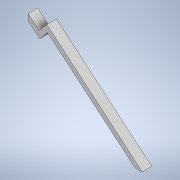
# Autodesk Inventor part: newFrame1x2piecsV03
Saved by Autodesk Inventor 2020.2 (Build 242310000, 310)
## iProperties
Created: 2020-02-22
Part Number: newFrame1x2piecsV03
Material: Generic
Document SubType Name: Modeling
Designer: robst
Density: 1 g/cm^3
Appearance: Default
Author: robst
Autodesk Inventor part; units mm, degrees
ref_plane "YZ Plane" through (0, 0, 0) normal (1, 0, 0) x (0, 1, 0)
ref_plane "XZ Plane" through (0, 0, 0) normal (0, 1, 0) x (-1, 0, 0)
ref_plane "XY Plane" through (0, 0, 0) normal (0, 0, 1) x (1, 0, 0)
sketch "Sketch1" plane through (0, 0, 0) normal (0, 0, 1) x (1, 0, 0)
  line L0 (0, 0) -> (-505.8958, 424.4969)
  line L1 (0, 0) -> (-228.6, 0) construction
  line L2 (0, 0) -> (-39.5154, 0)
  line L3 (-39.5154, 0) -> (-502.765, 388.7126)
  line L4 (-505.8958, 424.4969) -> (-522.2226, 405.0394)
  line L5 (-522.2226, 405.0394) -> (-546.7128, 375.8531)
  line L6 (-527.2552, 359.5263) -> (-502.765, 388.7126)
  line L7 (-546.7128, 375.8531) -> (-605.0854, 424.8335)
  line L8 (-605.0854, 391.6762) -> (-563.0396, 356.3956)
  line L9 (-543.582, 340.0688) -> (-527.2552, 359.5263)
  line L10 (-563.0396, 356.3956) -> (-543.582, 340.0688)
  line L11 (-228.6, 0) -> (-203.2, 0)
  line L12 (-605.0854, 424.8335) -> (-605.0854, 391.6762)
  line L13 (0, 0) -> (0, 391.6762) construction
  dimension "d2" = 660.4
  dimension "d3" = 25.4
  dimension "d4" = 40
  dimension "d25" = 50
  dimension "d34" = 63.5
  dimension "d35" = 76.2
  constraints: 28 end point, 3 perpendicular, 3 point on line, 2 collinear, 2 parallel, 2 vertical, 1 horizontal
  measures "d2" distance of L0.start L0.end
  measures "d3" distance between parallel lines of L3 L0
  measures "d4" angle of L3 L1
  measures "d25" angle of L12 L7
  measures "d34" distance from line of L9.start L3
  measures "d35" distance of L7.end L5.end
extrude "Extrusion1" add sketch "Sketch1" along normal mid plane 50.8
body "Solid1"
